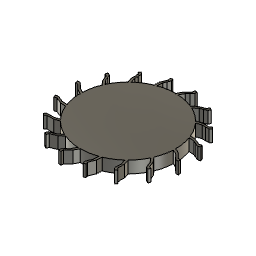
GearOdd (Autodesk Fusion 360 design; units mm, degrees)
Autodesk Fusion 360 part; units mm, degrees
sketch "Sketch1" plane through (0, 0, 0) normal (0, 0, 1) x (1, 0, 0)
  line L0 (0, 25.4) -> (1.27, 27.94)
  line L1 (1.27, 27.94) -> (2.54, 29.21)
  line L2 (2.54, 29.21) -> (3.81, 30.48)
  line L3 (3.81, 30.48) -> (3.81, 31.75)
  line L4 (3.81, 31.75) -> (5.08, 31.75)
  line L5 (5.08, 31.75) -> (5.08, 30.48)
  line L6 (5.08, 30.48) -> (3.81, 29.1148)
  line L7 (3.81, 29.1148) -> (2.54, 27.94)
  line L8 (2.54, 27.94) -> (1.778, 26.416)
  line L9 (1.778, 26.416) -> (1.2545, 25.369)
  arc A0 (1.2545, 25.369) -> (0, 25.4) centre (0, 0) ccw
  line L10 (-8.4663, 25.0856) -> (-8.5493, 23.918)
  line L11 (-8.8315, 27.9585) -> (-8.1442, 29.6179)
  arc A1 (-8.5493, 23.918) -> (-9.7202, 23.4665) centre (0, 0) ccw
  line L12 (-7.4569, 31.2772) -> (-6.9709, 30.1039)
  line L13 (-8.3455, 26.7852) -> (-8.4663, 25.0856)
  line L14 (-6.9709, 30.1039) -> (-7.6218, 28.3566)
  line L15 (-9.5188, 26.2992) -> (-8.8315, 27.9585)
  line L16 (-8.1442, 29.6179) -> (-8.6302, 30.7912)
  line L17 (-8.6302, 30.7912) -> (-7.4569, 31.2772)
  line L18 (-9.7202, 23.4665) -> (-9.5188, 26.2992)
  line L19 (-7.6218, 28.3566) -> (-8.3455, 26.7852)
  line L20 (-17.4217, 19.9362) -> (-17.0515, 18.8257)
  line L21 (-18.8585, 22.4506) -> (-18.8585, 24.2467)
  arc A2 (-17.0515, 18.8257) -> (-17.9605, 17.9605) centre (0, 0) ccw
  line L22 (-18.8585, 26.0427) -> (-17.9605, 25.1447)
  line L23 (-17.9605, 21.5526) -> (-17.4217, 19.9362)
  line L24 (-17.9605, 25.1447) -> (-17.8932, 23.2813)
  line L25 (-18.8585, 20.6546) -> (-18.8585, 22.4506)
  line L26 (-18.8585, 24.2467) -> (-19.7566, 25.1447)
  line L27 (-19.7566, 25.1447) -> (-18.8585, 26.0427)
  line L28 (-17.9605, 17.9605) -> (-18.8585, 20.6546)
  line L29 (-17.8932, 23.2813) -> (-17.9605, 21.5526)
  line L30 (-23.7248, 11.7516) -> (-22.9578, 10.8673)
  line L31 (-26.0145, 13.5248) -> (-26.7018, 15.1842)
  arc A3 (-22.9578, 10.8673) -> (-23.4665, 9.7202) centre (0, 0) ccw
  line L32 (-27.3891, 16.8435) -> (-26.2158, 16.3575)
  line L33 (-24.8412, 13.0388) -> (-23.7248, 11.7516)
  line L34 (-26.2158, 16.3575) -> (-25.4405, 14.6617)
  line L35 (-25.3272, 11.8655) -> (-26.0145, 13.5248)
  line L36 (-26.7018, 15.1842) -> (-27.8752, 15.6702)
  line L37 (-27.8752, 15.6702) -> (-27.3891, 16.8435)
  line L38 (-23.4665, 9.7202) -> (-25.3272, 11.8655)
  line L39 (-25.4405, 14.6617) -> (-24.8412, 13.0388)
  line L40 (-26.416, 1.778) -> (-25.369, 1.2545)
  line L41 (-29.21, 2.54) -> (-30.48, 3.81)
  arc A4 (-25.369, 1.2545) -> (-25.4, 0) centre (0, 0) ccw
  line L42 (-31.75, 5.08) -> (-30.48, 5.08)
  line L43 (-27.94, 2.54) -> (-26.416, 1.778)
  line L44 (-30.48, 5.08) -> (-29.1148, 3.81)
  line L45 (-27.94, 1.27) -> (-29.21, 2.54)
  line L46 (-30.48, 3.81) -> (-31.75, 3.81)
  line L47 (-31.75, 3.81) -> (-31.75, 5.08)
  line L48 (-25.4, 0) -> (-27.94, 1.27)
  line L49 (-29.1148, 3.81) -> (-27.94, 2.54)
  line L50 (-25.0856, -8.4663) -> (-23.918, -8.5493)
  line L51 (-27.9585, -8.8315) -> (-29.6179, -8.1442)
  arc A5 (-23.918, -8.5493) -> (-23.4665, -9.7202) centre (0, 0) ccw
  line L52 (-31.2772, -7.4569) -> (-30.1039, -6.9709)
  line L53 (-26.7852, -8.3455) -> (-25.0856, -8.4663)
  line L54 (-30.1039, -6.9709) -> (-28.3566, -7.6218)
  line L55 (-26.2992, -9.5188) -> (-27.9585, -8.8315)
  line L56 (-29.6179, -8.1442) -> (-30.7912, -8.6302)
  line L57 (-30.7912, -8.6302) -> (-31.2772, -7.4569)
  line L58 (-23.4665, -9.7202) -> (-26.2992, -9.5188)
  line L59 (-28.3566, -7.6218) -> (-26.7852, -8.3455)
  line L60 (-19.9362, -17.4217) -> (-18.8257, -17.0515)
  line L61 (-22.4506, -18.8585) -> (-24.2467, -18.8585)
  arc A6 (-18.8257, -17.0515) -> (-17.9605, -17.9605) centre (0, 0) ccw
  line L62 (-26.0427, -18.8585) -> (-25.1447, -17.9605)
  line L63 (-21.5526, -17.9605) -> (-19.9362, -17.4217)
  line L64 (-25.1447, -17.9605) -> (-23.2813, -17.8932)
  line L65 (-20.6546, -18.8585) -> (-22.4506, -18.8585)
  line L66 (-24.2467, -18.8585) -> (-25.1447, -19.7566)
  line L67 (-25.1447, -19.7566) -> (-26.0427, -18.8585)
  line L68 (-17.9605, -17.9605) -> (-20.6546, -18.8585)
  line L69 (-23.2813, -17.8932) -> (-21.5526, -17.9605)
  line L70 (-11.7516, -23.7248) -> (-10.8673, -22.9578)
  line L71 (-13.5248, -26.0145) -> (-15.1842, -26.7018)
  arc A7 (-10.8673, -22.9578) -> (-9.7202, -23.4665) centre (0, 0) ccw
  line L72 (-16.8435, -27.3891) -> (-16.3575, -26.2158)
  line L73 (-13.0388, -24.8412) -> (-11.7516, -23.7248)
  line L74 (-16.3575, -26.2158) -> (-14.6617, -25.4405)
  line L75 (-11.8655, -25.3272) -> (-13.5248, -26.0145)
  line L76 (-15.1842, -26.7018) -> (-15.6702, -27.8752)
  line L77 (-15.6702, -27.8752) -> (-16.8435, -27.3891)
  line L78 (-9.7202, -23.4665) -> (-11.8655, -25.3272)
  line L79 (-14.6617, -25.4405) -> (-13.0388, -24.8412)
  line L80 (-1.778, -26.416) -> (-1.2545, -25.369)
  line L81 (-2.54, -29.21) -> (-3.81, -30.48)
  arc A8 (-1.2545, -25.369) -> (0, -25.4) centre (0, 0) ccw
  line L82 (-5.08, -31.75) -> (-5.08, -30.48)
  line L83 (-2.54, -27.94) -> (-1.778, -26.416)
  line L84 (-5.08, -30.48) -> (-3.81, -29.1148)
  line L85 (-1.27, -27.94) -> (-2.54, -29.21)
  line L86 (-3.81, -30.48) -> (-3.81, -31.75)
  line L87 (-3.81, -31.75) -> (-5.08, -31.75)
  line L88 (0, -25.4) -> (-1.27, -27.94)
  line L89 (-3.81, -29.1148) -> (-2.54, -27.94)
  line L90 (8.4663, -25.0856) -> (8.5493, -23.918)
  line L91 (8.8315, -27.9585) -> (8.1442, -29.6179)
  arc A9 (8.5493, -23.918) -> (9.7202, -23.4665) centre (0, 0) ccw
  line L92 (7.4569, -31.2772) -> (6.9709, -30.1039)
  line L93 (8.3455, -26.7852) -> (8.4663, -25.0856)
  line L94 (6.9709, -30.1039) -> (7.6218, -28.3566)
  line L95 (9.5188, -26.2992) -> (8.8315, -27.9585)
  line L96 (8.1442, -29.6179) -> (8.6302, -30.7912)
  line L97 (8.6302, -30.7912) -> (7.4569, -31.2772)
  line L98 (9.7202, -23.4665) -> (9.5188, -26.2992)
  line L99 (7.6218, -28.3566) -> (8.3455, -26.7852)
  line L100 (17.4217, -19.9362) -> (17.0515, -18.8257)
  line L101 (18.8585, -22.4506) -> (18.8585, -24.2467)
  arc A10 (17.0515, -18.8257) -> (17.9605, -17.9605) centre (0, 0) ccw
  line L102 (18.8585, -26.0427) -> (17.9605, -25.1447)
  line L103 (17.9605, -21.5526) -> (17.4217, -19.9362)
  line L104 (17.9605, -25.1447) -> (17.8932, -23.2813)
  line L105 (18.8585, -20.6546) -> (18.8585, -22.4506)
  line L106 (18.8585, -24.2467) -> (19.7566, -25.1447)
  line L107 (19.7566, -25.1447) -> (18.8585, -26.0427)
  line L108 (17.9605, -17.9605) -> (18.8585, -20.6546)
  line L109 (17.8932, -23.2813) -> (17.9605, -21.5526)
  line L110 (23.7248, -11.7516) -> (22.9578, -10.8673)
  line L111 (26.0145, -13.5248) -> (26.7018, -15.1842)
  arc A11 (22.9578, -10.8673) -> (23.4665, -9.7202) centre (0, 0) ccw
  line L112 (27.3891, -16.8435) -> (26.2158, -16.3575)
  line L113 (24.8412, -13.0388) -> (23.7248, -11.7516)
  line L114 (26.2158, -16.3575) -> (25.4405, -14.6617)
  line L115 (25.3272, -11.8655) -> (26.0145, -13.5248)
  line L116 (26.7018, -15.1842) -> (27.8752, -15.6702)
  line L117 (27.8752, -15.6702) -> (27.3891, -16.8435)
  line L118 (23.4665, -9.7202) -> (25.3272, -11.8655)
  line L119 (25.4405, -14.6617) -> (24.8412, -13.0388)
  line L120 (26.416, -1.778) -> (25.369, -1.2545)
  line L121 (29.21, -2.54) -> (30.48, -3.81)
  arc A12 (25.369, -1.2545) -> (25.4, 0) centre (0, 0) ccw
  line L122 (31.75, -5.08) -> (30.48, -5.08)
  line L123 (27.94, -2.54) -> (26.416, -1.778)
  line L124 (30.48, -5.08) -> (29.1148, -3.81)
  line L125 (27.94, -1.27) -> (29.21, -2.54)
  line L126 (30.48, -3.81) -> (31.75, -3.81)
  line L127 (31.75, -3.81) -> (31.75, -5.08)
  line L128 (25.4, 0) -> (27.94, -1.27)
  line L129 (29.1148, -3.81) -> (27.94, -2.54)
  line L130 (25.0856, 8.4663) -> (23.918, 8.5493)
  line L131 (27.9585, 8.8315) -> (29.6179, 8.1442)
  arc A13 (23.918, 8.5493) -> (23.4665, 9.7202) centre (0, 0) ccw
  line L132 (31.2772, 7.4569) -> (30.1039, 6.9709)
  line L133 (26.7852, 8.3455) -> (25.0856, 8.4663)
  line L134 (30.1039, 6.9709) -> (28.3566, 7.6218)
  line L135 (26.2992, 9.5188) -> (27.9585, 8.8315)
  line L136 (29.6179, 8.1442) -> (30.7912, 8.6302)
  line L137 (30.7912, 8.6302) -> (31.2772, 7.4569)
  line L138 (23.4665, 9.7202) -> (26.2992, 9.5188)
  line L139 (28.3566, 7.6218) -> (26.7852, 8.3455)
  line L140 (19.9362, 17.4217) -> (18.8257, 17.0515)
  line L141 (22.4506, 18.8585) -> (24.2467, 18.8585)
  arc A14 (18.8257, 17.0515) -> (17.9605, 17.9605) centre (0, 0) ccw
  line L142 (26.0427, 18.8585) -> (25.1447, 17.9605)
  line L143 (21.5526, 17.9605) -> (19.9362, 17.4217)
  line L144 (25.1447, 17.9605) -> (23.2813, 17.8932)
  line L145 (20.6546, 18.8585) -> (22.4506, 18.8585)
  line L146 (24.2467, 18.8585) -> (25.1447, 19.7566)
  line L147 (25.1447, 19.7566) -> (26.0427, 18.8585)
  line L148 (17.9605, 17.9605) -> (20.6546, 18.8585)
  line L149 (23.2813, 17.8932) -> (21.5526, 17.9605)
  line L150 (11.7516, 23.7248) -> (10.8673, 22.9578)
  line L151 (13.5248, 26.0145) -> (15.1842, 26.7018)
  arc A15 (10.8673, 22.9578) -> (9.7202, 23.4665) centre (0, 0) ccw
  line L152 (16.8435, 27.3891) -> (16.3575, 26.2158)
  line L153 (13.0388, 24.8412) -> (11.7516, 23.7248)
  line L154 (16.3575, 26.2158) -> (14.6617, 25.4405)
  line L155 (11.8655, 25.3272) -> (13.5248, 26.0145)
  line L156 (15.1842, 26.7018) -> (15.6702, 27.8752)
  line L157 (15.6702, 27.8752) -> (16.8435, 27.3891)
  line L158 (9.7202, 23.4665) -> (11.8655, 25.3272)
  line L159 (14.6617, 25.4405) -> (13.0388, 24.8412)
  circle A16 centre (0, 0) radius 25.4
  dimension "d2" = 360
  constraint coincident A0.centre A1.centre
  constraint parallel L1 L2
  constraint vertical L3
  constraint perpendicular L3 L4
  constraint perpendicular L4 L5
  constraint parallel L8 L9
  constraint coincident L0.start A16
extrude "Extrude1" add sketch "Sketch1" along normal blind 6.35
